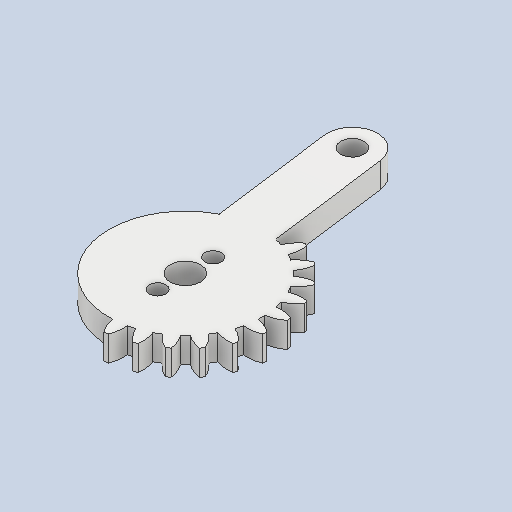
# Autodesk Inventor part: zubate_kolo2
Saved by Autodesk Inventor 2023 (Build 270158000, 158)
## iProperties
Part Number: zubate_kolo2
Material: ABS Plastic
Document SubType Name: Modeling
Designer: denyh
Density: 1.06 g/cm^3
Appearance: Smooth - White
Mass: 2.71646 g
Surface Area: 21.0316 cm^2
Volume: 2.5627 cm^3
Author: denyh
Autodesk Inventor part; units mm, degrees
ref_plane "YZ Plane" through (0, 0, 0) normal (1, 0, 0) x (0, 1, 0)
ref_plane "XZ Plane" through (0, 0, 0) normal (0, 1, 0) x (-1, 0, 0)
ref_plane "XY Plane" through (0, 0, 0) normal (0, 0, 1) x (1, 0, 0)
sketch "Náčrt1" plane through (0, 0, 0) normal (0, 0, 1) x (1, 0, 0)
  circle A0 centre (0, 0) radius 12.0945
  line L0 (0, 0) -> (0.5842, 13.9377)
  arc A1 (5.5661, 10.7376) -> (5.8875, 13.3827) centre (0.5319, 12.6914) ccw
  arc A2 (8.1555, 8.9311) -> (9.1506, 11.4029) centre (3.7986, 12.1212) ccw
  arc A3 (10.1892, 6.516) -> (11.7901, 8.646) centre (6.8063, 10.7251) ccw
  arc A4 (11.5284, 3.6568) -> (13.6261, 5.2999) centre (9.3503, 8.598) ccw
  arc A5 (12.0821, 0.5484) -> (14.5335, 1.5926) centre (11.257, 5.885) ccw
  arc A6 (11.8123, -2.5973) -> (14.4505, -2.2232) centre (12.3966, 2.771) ccw
  arc A7 (10.7376, -5.5661) -> (13.3827, -5.8875) centre (12.6914, -0.5319) ccw
  arc A8 (8.9311, -8.1555) -> (11.4029, -9.1506) centre (12.1212, -3.7986) ccw
  arc A9 (6.516, -10.1892) -> (8.646, -11.7901) centre (10.7251, -6.8063) ccw
  arc A10 (3.6568, -11.5284) -> (5.2999, -13.6261) centre (8.598, -9.3503) ccw
  arc A11 (0.5484, -12.0821) -> (1.5926, -14.5335) centre (5.885, -11.257) ccw
  line L1 (0, 0) -> (0, 15.3936)
  arc A12 (5.2999, 13.6261) -> (3.6568, 11.5284) centre (8.598, 9.3503) ccw
  arc A13 (8.646, 11.7901) -> (6.516, 10.1892) centre (10.7251, 6.8063) ccw
  arc A14 (11.4029, 9.1506) -> (8.9311, 8.1555) centre (12.1212, 3.7986) ccw
  arc A15 (13.3827, 5.8875) -> (10.7376, 5.5661) centre (12.6914, 0.5319) ccw
  arc A16 (14.4505, 2.2232) -> (11.8123, 2.5973) centre (12.3966, -2.771) ccw
  arc A17 (14.5335, -1.5926) -> (12.0821, -0.5484) centre (11.257, -5.885) ccw
  arc A18 (13.6261, -5.2999) -> (11.5284, -3.6568) centre (9.3503, -8.598) ccw
  arc A19 (11.7901, -8.646) -> (10.1892, -6.516) centre (6.8063, -10.7251) ccw
  arc A20 (9.1506, -11.4029) -> (8.1555, -8.9311) centre (3.7986, -12.1212) ccw
  arc A21 (5.8875, -13.3827) -> (5.5661, -10.7376) centre (0.5319, -12.6914) ccw
  arc A22 (2.2232, -14.4505) -> (2.5973, -11.8123) centre (-2.771, -12.3966) ccw
  arc A23 (5.8875, 13.3827) -> (5.2999, 13.6261) centre (0, 0) ccw
  arc A24 (9.1506, 11.4029) -> (8.646, 11.7901) centre (0, 0) ccw
  arc A25 (11.7901, 8.646) -> (11.4029, 9.1506) centre (0, 0) ccw
  arc A26 (13.6261, 5.2999) -> (13.3827, 5.8875) centre (0, 0) ccw
  arc A27 (14.5335, 1.5926) -> (14.4505, 2.2232) centre (0, 0) ccw
  arc A28 (14.4505, -2.2232) -> (14.5335, -1.5926) centre (0, 0) ccw
  arc A29 (13.3827, -5.8875) -> (13.6261, -5.2999) centre (0, 0) ccw
  arc A30 (11.4029, -9.1506) -> (11.7901, -8.646) centre (0, 0) ccw
  arc A31 (8.646, -11.7901) -> (9.1506, -11.4029) centre (0, 0) ccw
  arc A32 (1.5926, -14.5335) -> (2.2232, -14.4505) centre (0, 0) ccw
  arc A33 (5.2999, -13.6261) -> (5.8875, -13.3827) centre (0, 0) ccw
  dimension "d0" = 24.189
  dimension "d13" = 150
  dimension "d19" = 150
  constraints: 68 point on circle, 34 centre point, 4 end point, 3 coincident, 1 point on line, 1 vertical, 82 other
  measures "d0" diameter of A0
sketch "Náčrt2" plane through (0, 0, 0) normal (0, 0, 1) x (1, 0, 0)
  circle A0 centre (0, 0) radius 12.0945 projected
  circle A1 centre (0, 0) radius 12.0945
  constraints: 1 centre point, 1 coincident, 1 concentric
extrude "Vysunutí1" add sketch "Náčrt2" along normal blind 4
extrude "Vysunutí2" add sketch "Náčrt1" along normal blind 4 contours A0 A12 A23 A1
pattern_circular "Kruhové pole1" count 11 over 150 about axis through (0, 0, 0) along (0, 0, -1) of "Vysunutí2"
sketch "Náčrt3" plane through (0, 0, 4) normal (0, 0, 1) x (1, 0, 0)
  line L0 (0, 0) -> (-4.0046, 30.5002)
  circle A0 centre (-4.0046, 30.5002) radius 1.825
  arc A1 (-0.0386, 31.0209) -> (-7.9706, 29.9795) centre (-4.0046, 30.5002) ccw
  line L1 (-3.966, -0.5207) -> (-7.9706, 29.9795)
  line L2 (3.966, 0.5207) -> (-0.0386, 31.0209)
  line L3 (-5.0618, 7.8256) -> (2.8701, 8.867)
  dimension "d29" = 30.762
  dimension "d30" = 3.65
  dimension "d31" = 8
  dimension "d32" = 4
  dimension "d33" = 4
  constraints: 8 end point, 2 centre point, 2 coincident, 2 parallel, 2 point on circle, 2 point on line, 1 perpendicular
  measures "d29" distance of L0.start L0.end
  measures "d30" diameter of A0
  measures "d31" diameter of A1
  measures "d32" distance between parallel lines of L0 L1
  measures "d33" distance between parallel lines of L0 L2
extrude "Vysunutí3" add sketch "Náčrt3" against normal blind 4
sketch "Náčrt4" plane through (0, 0, 4) normal (0, 0, 1) x (1, 0, 0)
  circle A0 centre (0, 0) radius 2.4
  line L0 (0, 0) -> (0, -4.4)
  circle A1 centre (0, -4.4) radius 1.3
  line L1 (0, 0) -> (0, 4.4)
  circle A2 centre (0, 4.4) radius 1.3
  dimension "d36" = 4.8
  dimension "d37" = 4.4
  dimension "d38" = 2.6
  dimension "d39" = 4.4
  dimension "d40" = 2.6
  constraints: 4 end point, 3 centre point, 3 coincident, 2 vertical
  measures "d36" diameter of A0
  measures "d37" distance of L0.start L0.end
  measures "d38" diameter of A1
  measures "d39" distance of L0.start L1.end
  measures "d40" diameter of A2
extrude "Vysunutí4" cut sketch "Náčrt4" against normal blind 4
